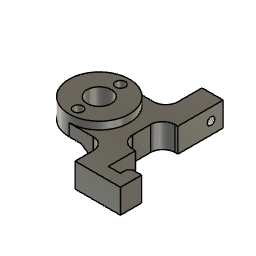
headcamera_arm1 (Autodesk Fusion 360 design; units mm, degrees)
Autodesk Fusion 360 part; units mm, degrees
sketch "スケッチ1" plane through (0, 0, 0) normal (0, 0, 1) x (1, 0, 0)
  circle A0 centre (0, 0) radius 10
  line L0 (0, 10) -> (12, 10)
  line L1 (12, 10) -> (12, 22)
  line L2 (19, 22) -> (19, -16)
  line L3 (12, -20) -> (12, -10)
  line L4 (12, -10) -> (0, -10)
  line L5 (0, -7) -> (0, 7)
  line L6 (19, -7) -> (14, -7)
  line L7 (14, -7) -> (14, 7)
  line L8 (14, 7) -> (19, 7)
  line L9 (12, 22) -> (19, 22)
  line L10 (12, -20) -> (27, -20)
  line L11 (27, -20) -> (27, -13)
  line L12 (27, -13) -> (23, -13)
  line L13 (23, -13) -> (23, -16)
  line L14 (23, -16) -> (19, -16)
  point P0 (14, 0)
  dimension "d1" = 20
  dimension "d2" = 12
  dimension "d6" = 7
  dimension "d19" = 14
  dimension "d31" = 5
  dimension "d32" = 14
  dimension "d39" = 22
  dimension "d40" = 13
  dimension "d41" = 3
  dimension "d42" = 4
  dimension "d43" = 4
  dimension "d44" = 4
  constraint coincident A0.centre origin
  constraint coincident A0 L0.start
  constraint horizontal L0
  constraint perpendicular L0 L1
  constraint coincident A0 L4.end
  constraint perpendicular L2 L4
  constraint tangent A0 L0
  constraint tangent A0 L4
  constraint collinear L1 L3
  constraint midpoint A0.centre L5
  constraint vertical L5
  constraint coincident L2 L6.start
  constraint perpendicular L2 L6
  constraint perpendicular L6 L7
  constraint coincident L2 L8.end
  constraint perpendicular L2 L8
  constraint midpoint L7 P0
  constraint horizontal A0.centre P0
  constraint perpendicular L1 L9
  constraint coincident L2.start L9.end
  constraint perpendicular L3 L10
  constraint perpendicular L10 L11
  constraint perpendicular L11 L12
  constraint perpendicular L12 L13
  constraint perpendicular L2 L14
  constraint coincident L2.end L14.end
  measures "d1" diameter of A0
  measures "d2" distance of A0.centre L1
  measures "d6" distance of L1 L2
  measures "d19" distance of L5.start L5.end
  measures "d31" distance of L6.start L6.end
  measures "d32" distance of L6 L8
  measures "d39" distance of A0.centre L9
  measures "d40" distance of A0.centre L12
  measures "d41" distance of L12 L14
  measures "d42" distance of L10 L14
  measures "d43" distance of L2 L13
  measures "d44" distance of L11.end L12.end
extrude "押し出し1" add sketch "スケッチ1" along normal blind 8 contours A0 | A0 L0 L1 L2 L3 L4 L6 L7 L8 L9 L10 L11 L12 L13 L14
sketch "スケッチ2" plane through (0, 0, 8) normal (0, 0, 1) x (-1, 0, 0)
  circle A0 centre (0, 0) radius 10
  line L0 (-12, 20) -> (-27, 20)
  line L1 (-27, 20) -> (-27, 13)
  line L2 (-27, 13) -> (-23, 13)
  line L3 (-23, 13) -> (-23, 16)
  line L4 (-23, 16) -> (-19, 16)
  line L5 (-19, 16) -> (-19, 7)
  line L6 (-19, -22) -> (-12, -22)
  line L7 (-12, -22) -> (-12, -10)
  line L8 (-12, -10) -> (0, -10)
  arc A1 (0, -10) -> (0, 10) centre (0, 0) ccw
  line L9 (0, 10) -> (-12, 10)
  line L10 (-12, 10) -> (-12, 20)
  line L11 (-19, 7) -> (-14, 7)
  line L12 (-14, 7) -> (-14, -7)
  line L13 (-14, -7) -> (-19, -7)
  line L14 (-19, -7) -> (-19, -22)
  constraint coincident A0 L8.end
  constraint coincident A0.centre A1.centre
extrude "押し出し2" add sketch "スケッチ2" along normal blind 2.5 contours A0 A1
hole "穴1" at (0, 7, 0) at (0, -7, 0) direction (0, 0, 1) diameter 3.2 end through all
hole "穴3" at (0, 0, 0) direction (0, 0, 1) diameter 8 end through all
sketch "スケッチ3" plane through (0, -10, 0) normal (0, -1, 0) x (1, 0, 0)
  line L0 (0, 0) -> (12, 0)
  line L1 (12, 0) -> (12, 8)
  line L2 (12, 8) -> (0, 8)
  line L3 (0, 8) -> (0, 0)
  line L4 (10, 0) -> (4, 4)
  line L5 (4, 4) -> (-15, 4)
  line L6 (-15, 4) -> (-15, 0)
  line L7 (-15, 0) -> (10, 0)
  dimension "d20" = 10
  dimension "d21" = 15
  dimension "d22" = 6
  dimension "d23" = 4
  constraint coincident L0 L4.start
  constraint parallel L0 L5
  constraint perpendicular L5 L6
  constraint perpendicular L6 L7
  measures "d20" distance of L0.start L4.start
  measures "d21" distance of L0.start L6
  measures "d22" horizontal distance of L4.start L4.end
  measures "d23" vertical distance of L4.start L4.end
extrude "押し出し3" cut sketch "スケッチ3" against normal through all contours L0 L3 L4 L5 L7 | L3 L5 L6 L7
sketch "スケッチ4" plane through (19, 0, 0) normal (1, 0, 0) x (0, 1, 0)
  line L0 (7, 0) -> (22, 0)
  line L1 (22, 8) -> (7, 8)
  line L2 (22, 4) -> (18, 4)
  line L3 (22, 0) -> (22, 8)
  line L4 (-16, 8) -> (-16, 0)
  line L5 (7, 8) -> (7, 0)
  line L6 (-16, 0) -> (-7, 0)
  line L7 (-7, 0) -> (-7, 8)
  line L8 (-7, 8) -> (-16, 8)
  dimension "d45" = 4
  constraint midpoint L2.start L3
  constraint horizontal L2
  measures "d45" distance of L2.start L2.end
hole "穴2" at (19, 18, 4) direction (-1, 0, 0) diameter 3 depth 11 tip angle 118
thread "ねじ1" "ISO Metric profile 3.0 M3x0.5 6H" major diameter 3.086 minor diameter 2.529 pitch 0.5 angle 60 resizes the face on face at (16.6667, 18.0748, 2.5019)
fillet "フィレット1" radius 4 4 edges at (12, 10, 4) (12, -10, 4) (14, -7, 4) (14, 7, 4)
chamfer "面取り2" distance 1 angle 45 1 edges at (23, -13, 4)
